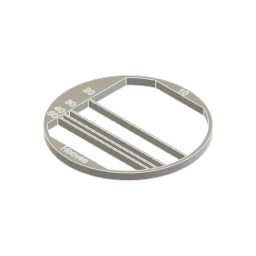
Range Finder-White Tail Deer v3 (Autodesk Fusion 360 design; units mm, degrees)
Autodesk Fusion 360 part; units mm, degrees
sketch "Sketch1" plane through (0, 0, 0) normal (0, 1, 0) x (1, 0, 0)
  circle A0 centre (0, 0) radius 57.15
  circle A1 centre (0, 0) radius 54.61
  dimension "d1" = 114.3
  dimension "d2" = 109.22
  constraint coincident A0.centre A1.centre
  constraint concentric A0 A1
  measures "d1" diameter of A0
  measures "d2" diameter of A1
extrude "Extrude1" add sketch "Sketch1" along normal blind 6.35
sketch "Sketch2" plane through (0, 6.35, 0) normal (0, 1, 0) x (-1, 0, 0)
  circle A0 centre (0, 0) radius 54.61
  circle A1 centre (0, 0) radius 57.15
  line L0 (0, 54.61) -> (0, 46.99)
  line L1 (0, 46.99) -> (27.8243, 46.99)
  line L2 (-27.8243, 46.99) -> (0, 46.99)
  dimension "d5" = 7.62
  constraint coincident A0 L0.start
  constraint vertical L0
  constraint coincident A0 L1.end
  constraint perpendicular L0 L1
  constraint coincident A0 L2.start
  constraint perpendicular L0 L2
  measures "d5" distance of L0.start L0.end
extrude "Extrude2" add sketch "Sketch2" against normal blind 6.35 contours A0 L0 L1 | A0 L0 L2
sketch "Sketch3" plane through (0, 6.35, 0) normal (0, 1, 0) x (-1, 0, 0)
  arc A0 (-27.8243, 46.99) -> (27.8243, 46.99) centre (0, 0) ccw
  line L0 (-27.8243, 46.99) -> (27.8243, 46.99)
  circle A1 centre (0, 0) radius 57.15
  line L1 (0, -49.53) -> (23.0007, -49.53)
  line L2 (0, -49.53) -> (-23.0007, -49.53)
  arc A2 (-23.0007, -49.53) -> (23.0007, -49.53) centre (0, 0) ccw
  line L3 (54.5858, -1.6242) -> (-54.5952, -1.27)
  line L4 (-52.0545, 16.51) -> (52.0545, 16.51)
  line L5 (0, 22.86) -> (49.5951, 22.86)
  line L6 (0, 22.86) -> (-49.5951, 22.86)
  line L7 (0, 27.686) -> (47.0716, 27.686)
  line L8 (0, 27.686) -> (-47.0716, 27.686)
  line L9 (0, 27.686) -> (0, 26.416)
  line L10 (0, 22.86) -> (0, 21.59)
  line L11 (0, 16.51) -> (0, 15.24)
  line L12 (-0.0047, -1.4471) -> (-0.0088, -2.7171)
  line L13 (-0.0088, -2.7171) -> (54.5333, -2.894)
  line L14 (-0.0088, -2.7171) -> (-54.5509, -2.5402)
  line L15 (0, 15.24) -> (52.4404, 15.24)
  line L16 (0, 15.24) -> (-52.4404, 15.24)
  line L17 (0, 21.59) -> (-50.161, 21.59)
  line L18 (0, 21.59) -> (50.161, 21.59)
  line L19 (0, 26.416) -> (47.7959, 26.416)
  line L20 (0, 26.416) -> (-47.7959, 26.416)
  dimension "d16" = 1.27
  dimension "d17" = 1.27
  dimension "d18" = 1.27
  dimension "d19" = 1.27
  constraint coincident A0 L1.end
  constraint coincident A0 L2.end
  constraint coincident A0 L3.end
  constraint coincident A0 L3.start
  constraint coincident A0 L4.end
  constraint coincident A0 L4.start
  constraint horizontal L4
  constraint coincident A0 L5.end
  constraint coincident A0 L6.end
  constraint coincident A0 L7.end
  constraint coincident A0 L8.end
  constraint perpendicular L7 L9
  constraint perpendicular L6 L10
  constraint midpoint L4 L11.start
  constraint perpendicular L4 L11
  constraint midpoint L3 L12.start
  constraint perpendicular L3 L12
  constraint coincident A0 L13.end
  constraint perpendicular L12 L13
  constraint coincident A0 L14.end
  constraint perpendicular L12 L14
  constraint coincident A0 L15.end
  constraint perpendicular L11 L15
  constraint coincident A0 L16.end
  constraint perpendicular L11 L16
  constraint coincident A0 L17.end
  constraint perpendicular L10 L17
  constraint coincident A0 L18.end
  constraint perpendicular L10 L18
  constraint coincident A0 L19.end
  constraint perpendicular L9 L19
  constraint perpendicular L9 L20
  constraint coincident A0 L20.end
  constraint horizontal L20
  measures "d16" distance of L7.start L9.end
  measures "d17" distance of L5.start L10.end
  measures "d18" distance of L11.start L11.end
  measures "d19" distance of L12.start L12.end
extrude "Extrude3" add sketch "Sketch3" against normal blind 6.35 contours A0 L8 L9 L20 | A0 L7 L9 L19 | A0 L6 L10 L17 | A0 L5 L10 L18 | A0 L4 L11 L16 | A0 L4 L11 L15 | A0 L3 L12 L14 | A0 L3 L12 L13 | A0 L1 L2 A2
sketch "Sketch4" plane through (0, 6.35, 0) normal (0, 1, 0) x (-1, 0, 0)
  arc A0 (-52.4404, 15.24) -> (-54.5952, -1.27) centre (0, 0) ccw
  line L0 (-52.4404, 15.24) -> (52.4404, 15.24)
  arc A1 (54.5858, -1.6242) -> (52.4404, 15.24) centre (0, 0) ccw
  line L1 (54.5858, -1.6242) -> (-54.5952, -1.27)
  arc A2 (-27.8243, 46.99) -> (-47.0716, 27.686) centre (0, 0) ccw
  line L2 (-27.8243, 46.99) -> (27.8243, 46.99)
  arc A3 (47.0716, 27.686) -> (27.8243, 46.99) centre (0, 0) ccw
  line L3 (47.0716, 27.686) -> (-47.0716, 27.686)
  arc A4 (-50.161, 21.59) -> (-52.0545, 16.51) centre (0, 0) ccw
  line L4 (-50.161, 21.59) -> (50.161, 21.59)
  arc A5 (52.0545, 16.51) -> (50.161, 21.59) centre (0, 0) ccw
  line L5 (52.0545, 16.51) -> (-52.0545, 16.51)
  line L6 (-47.7959, 26.416) -> (47.7959, 26.416)
  arc A6 (49.5951, 22.86) -> (47.7959, 26.416) centre (0, 0) ccw
  line L7 (49.5951, 22.86) -> (-49.5951, 22.86)
  arc A7 (-47.7959, 26.416) -> (-49.5951, 22.86) centre (0, 0) ccw
  line L8 (-54.5509, -2.5402) -> (54.5333, -2.894)
  arc A8 (23.0007, -49.53) -> (54.5333, -2.894) centre (0, 0) ccw
  line L9 (23.0007, -49.53) -> (-23.0007, -49.53)
  arc A9 (-54.5509, -2.5402) -> (-23.0007, -49.53) centre (0, 0) ccw
  circle A10 centre (0, 0) radius 57.15
  line L10 (20.3865, 53.4838) -> (-20.1396, 53.4838) construction
  line L11 (-20.1396, 53.4838) -> (-20.1396, 46.99) construction
  line L12 (-20.1396, 46.99) -> (20.3865, 46.99) construction
  line L13 (20.3865, 46.99) -> (20.3865, 53.4838) construction
  line L14 (6.9725, -49.53) -> (-6.8843, -49.53) construction
  line L15 (-6.8843, -49.53) -> (-6.8843, -56.7231) construction
  line L16 (-6.8843, -56.7231) -> (6.9725, -56.7231) construction
  line L17 (6.9725, -56.7231) -> (6.9725, -49.53) construction
  dimension "d22" = 5.08
  dimension "d24" = 5.08
  dimension "d25" = 0
  text T0 "Hooves" font "Arial" height 5.08 align centre middle in box 40.5261 x 6.4938 at (20.3865, 53.4838) x (-1, 0) y (0, -1) spacing 1
  text T1 "10" font "Arial" height 5.08 align centre middle in box 13.8568 x 7.1931 at (6.9725, -49.53) x (-1, 0) y (0, -1) spacing 1
  constraint coincident A10
  constraint coincident L2
  constraint coincident L9
extrude "Extrude4" cut sketch "Sketch4" against normal blind 1.27 text T1 T0
sketch "Sketch5" plane through (0, 6.35, 0) normal (0, 1, 0) x (-1, 0, 0)
  spline S0 degree 3 poles (5.2156, 52.8601) (5.458, 52.8423) (5.9273, 52.8079) (6.2896, 52.509) (6.4648, 52.3645) knots 0 0 0 0 0.070957 0.137381 0.137381 0.137381 0.137381
  spline S1 degree 3 poles (6.4648, 52.3645) (6.6035, 52.1699) (6.9064, 51.7448) (6.929, 51.2209) (6.9412, 50.9369) knots 0 0 0 0 0.070238 0.153394 0.153394 0.153394 0.153394
  spline S2 degree 3 poles (6.9412, 50.9369) (6.927, 50.6271) (6.9009, 50.0574) (6.5384, 49.6215) (6.3729, 49.4226) knots 0 0 0 0 0.090097 0.165714 0.165714 0.165714 0.165714
  spline S3 degree 3 poles (6.3729, 49.4226) (6.2035, 49.3033) (5.8563, 49.0591) (5.4325, 49.0291) (5.2156, 49.0137) knots 0 0 0 0 0.060949 0.124839 0.124839 0.124839 0.124839
  spline S4 degree 3 poles (5.2156, 49.0137) (4.9764, 49.0322) (4.51, 49.0682) (4.1502, 49.3659) (3.975, 49.5109) knots 0 0 0 0 0.070069 0.136601 0.136601 0.136601 0.136601
  spline S5 degree 3 poles (3.975, 49.5109) (3.8347, 49.701) (3.5343, 50.1079) (3.5076, 50.6148) (3.4934, 50.8849) knots 0 0 0 0 0.069362 0.148467 0.148467 0.148467 0.148467
  spline S6 degree 3 poles (3.4934, 50.8849) (3.4975, 51.0992) (3.505, 51.4847) (3.6445, 51.8432) (3.7065, 52.0024) knots 0 0 0 0 0.06368 0.114552 0.114552 0.114552 0.114552
  spline S7 degree 3 poles (3.7065, 52.0024) (3.7858, 52.1307) (3.945, 52.3881) (4.1992, 52.5524) (4.3267, 52.6348) knots 0 0 0 0 0.044639 0.089574 0.089574 0.089574 0.089574
  spline S8 degree 3 poles (4.3267, 52.6348) (4.4663, 52.7005) (4.7479, 52.8331) (5.0587, 52.851) (5.2156, 52.8601) knots 0 0 0 0 0.045807 0.092452 0.092452 0.092452 0.092452
  spline S9 degree 3 poles (-10.0036, 52.8601) (-9.7875, 52.854) (-9.3973, 52.843) (-9.0606, 52.6487) (-8.9104, 52.5621) knots 0 0 0 0 0.063634 0.114894 0.114894 0.114894 0.114894
  spline S10 degree 3 poles (-8.9104, 52.5621) (-8.7955, 52.4455) (-8.5515, 52.1979) (-8.4723, 51.8583) (-8.4304, 51.6784) knots 0 0 0 0 0.048133 0.102307 0.102307 0.102307 0.102307
  line L0 (-8.4304, 51.6784) -> (-9.0472, 51.5814)
  spline S11 degree 3 poles (-9.0472, 51.5814) (-9.07, 51.6958) (-9.1132, 51.913) (-9.2648, 52.0737) (-9.3366, 52.1497) knots 0 0 0 0 0.034191 0.06493 0.06493 0.06493 0.06493
  spline S12 degree 3 poles (-9.3366, 52.1497) (-9.4289, 52.2072) (-9.6312, 52.3332) (-9.8702, 52.3423) (-10.0002, 52.3472) knots 0 0 0 0 0.032083 0.070304 0.070304 0.070304 0.070304
  spline S13 degree 3 poles (-10.0002, 52.3472) (-10.1284, 52.3443) (-10.3567, 52.339) (-10.5521, 52.2231) (-10.6378, 52.1722) knots 0 0 0 0 0.037679 0.067104 0.067104 0.067104 0.067104
  spline S14 degree 3 poles (-10.6378, 52.1722) (-10.6984, 52.1131) (-10.8148, 51.9995) (-10.8357, 51.8387) (-10.8457, 51.7616) knots 0 0 0 0 0.024591 0.047243 0.047243 0.047243 0.047243
  spline S15 degree 3 poles (-10.8457, 51.7616) (-10.8377, 51.6947) (-10.8214, 51.5591) (-10.7156, 51.4727) (-10.662, 51.4289) knots 0 0 0 0 0.019436 0.039349 0.039349 0.039349 0.039349
  spline S16 degree 3 poles (-10.662, 51.4289) (-10.5881, 51.3958) (-10.3832, 51.3037) (-10.1644, 51.2512) (-10.0244, 51.2176) knots 0 0 0 0 0.024263 0.067292 0.067292 0.067292 0.067292
  spline S17 degree 3 poles (-10.0244, 51.2176) (-9.8292, 51.1687) (-9.506, 51.0877) (-9.196, 50.966) (-9.0732, 50.9178) knots 0 0 0 0 0.060291 0.099819 0.099819 0.099819 0.099819
  spline S18 degree 3 poles (-9.0732, 50.9178) (-8.991, 50.8728) (-8.8312, 50.7854) (-8.7235, 50.6389) (-8.6713, 50.5678) knots 0 0 0 0 0.027754 0.053876 0.053876 0.053876 0.053876
  spline S19 degree 3 poles (-8.6713, 50.5678) (-8.6314, 50.491) (-8.5509, 50.3361) (-8.5399, 50.1619) (-8.5344, 50.074) knots 0 0 0 0 0.025663 0.051747 0.051747 0.051747 0.051747
  spline S20 degree 3 poles (-8.5344, 50.074) (-8.5389, 49.9939) (-8.5479, 49.8349) (-8.6142, 49.6901) (-8.647, 49.6184) knots 0 0 0 0 0.02386 0.047308 0.047308 0.047308 0.047308
  spline S21 degree 3 poles (-8.647, 49.6184) (-8.688, 49.5514) (-8.7699, 49.4175) (-8.8924, 49.3193) (-8.9537, 49.2701) knots 0 0 0 0 0.023346 0.046717 0.046717 0.046717 0.046717
  spline S22 degree 3 poles (-8.9537, 49.2701) (-9.0099, 49.2347) (-9.134, 49.1567) (-9.2739, 49.1124) (-9.3505, 49.0882) knots 0 0 0 0 0.019852 0.043806 0.043806 0.043806 0.043806
  spline S23 degree 3 poles (-9.3505, 49.0882) (-9.4368, 49.0665) (-9.6137, 49.022) (-9.796, 49.0165) (-9.8893, 49.0137) knots 0 0 0 0 0.026625 0.054539 0.054539 0.054539 0.054539
  spline S24 degree 3 poles (-9.8893, 49.0137) (-10.026, 49.0177) (-10.2853, 49.0252) (-10.5328, 49.1021) (-10.6499, 49.1384) knots 0 0 0 0 0.040792 0.077397 0.077397 0.077397 0.077397
  spline S25 degree 3 poles (-10.6499, 49.1384) (-10.7496, 49.1807) (-10.9351, 49.2592) (-11.0706, 49.4076) (-11.1333, 49.4763) knots 0 0 0 0 0.032023 0.059594 0.059594 0.059594 0.059594
  spline S26 degree 3 poles (-11.1333, 49.4763) (-11.1819, 49.5575) (-11.2876, 49.7343) (-11.3269, 49.9368) (-11.3482, 50.0463) knots 0 0 0 0 0.028173 0.061329 0.061329 0.061329 0.061329
  line L1 (-11.3482, 50.0463) -> (-10.7383, 50.1295)
  spline S27 degree 3 poles (-10.7383, 50.1295) (-10.719, 50.0409) (-10.6817, 49.8694) (-10.5575, 49.7457) (-10.4974, 49.6859) knots 0 0 0 0 0.026561 0.051435 0.051435 0.051435 0.051435
  spline S28 degree 3 poles (-10.4974, 49.6859) (-10.4193, 49.6396) (-10.2464, 49.537) (-10.0448, 49.5302) (-9.9343, 49.5265) knots 0 0 0 0 0.026848 0.059363 0.059363 0.059363 0.059363
  spline S29 degree 3 poles (-9.9343, 49.5265) (-9.8088, 49.5276) (-9.5926, 49.5293) (-9.4013, 49.6274) (-9.321, 49.6686) knots 0 0 0 0 0.036989 0.063721 0.063721 0.063721 0.063721
  spline S30 degree 3 poles (-9.321, 49.6686) (-9.2675, 49.716) (-9.1663, 49.8055) (-9.1466, 49.9386) (-9.1373, 50.0013) knots 0 0 0 0 0.020676 0.039103 0.039103 0.039103 0.039103
  spline S31 degree 3 poles (-9.1373, 50.0013) (-9.1406, 50.0408) (-9.1471, 50.1201) (-9.1913, 50.1863) (-9.2136, 50.2196) knots 0 0 0 0 0.011678 0.023467 0.023467 0.023467 0.023467
  spline S32 degree 3 poles (-9.2136, 50.2196) (-9.2446, 50.2524) (-9.3126, 50.3243) (-9.4034, 50.3642) (-9.4527, 50.3859) knots 0 0 0 0 0.013422 0.029388 0.029388 0.029388 0.029388
  spline S33 degree 3 poles (-9.4527, 50.3859) (-9.5141, 50.4053) (-9.6965, 50.4627) (-9.8812, 50.5124) (-10.0036, 50.5453) knots 0 0 0 0 0.019318 0.057361 0.057361 0.057361 0.057361
  spline S34 degree 3 poles (-10.0036, 50.5453) (-10.192, 50.5953) (-10.5042, 50.6782) (-10.8071, 50.7903) (-10.9271, 50.8347) knots 0 0 0 0 0.058433 0.096821 0.096821 0.096821 0.096821
  spline S35 degree 3 poles (-10.9271, 50.8347) (-11.009, 50.8756) (-11.1693, 50.9557) (-11.2824, 51.0944) (-11.3378, 51.1621) knots 0 0 0 0 0.027129 0.053055 0.053055 0.053055 0.053055
  spline S36 degree 3 poles (-11.3378, 51.1621) (-11.3812, 51.2406) (-11.4729, 51.4064) (-11.482, 51.596) (-11.4868, 51.6958) knots 0 0 0 0 0.02655 0.056067 0.056067 0.056067 0.056067
  spline S37 degree 3 poles (-11.4868, 51.6958) (-11.4787, 51.7989) (-11.4624, 52.0083) (-11.3579, 52.1906) (-11.3048, 52.2831) knots 0 0 0 0 0.030617 0.062177 0.062177 0.062177 0.062177
  spline S38 degree 3 poles (-11.3048, 52.2831) (-11.2357, 52.3705) (-11.0925, 52.5514) (-10.8864, 52.6555) (-10.7799, 52.7093) knots 0 0 0 0 0.033024 0.068346 0.068346 0.068346 0.068346
  spline S39 degree 3 poles (-10.7799, 52.7093) (-10.6592, 52.7533) (-10.4086, 52.8446) (-10.142, 52.8548) (-10.0036, 52.8601) knots 0 0 0 0 0.038266 0.079502 0.079502 0.079502 0.079502
  spline S40 degree 3 poles (-6.282, 52.3472) (-6.3907, 52.3408) (-6.6008, 52.3284) (-6.7808, 52.2196) (-6.8676, 52.167) knots 0 0 0 0 0.032111 0.062098 0.062098 0.062098 0.062098
  spline S41 degree 3 poles (-6.8676, 52.167) (-6.946, 52.0931) (-7.1175, 51.9311) (-7.2048, 51.7113) (-7.2523, 51.5918) knots 0 0 0 0 0.031936 0.069943 0.069943 0.069943 0.069943
  line L2 (-7.2523, 51.5918) -> (-7.8968, 51.6715)
  spline S42 degree 3 poles (-7.8968, 51.6715) (-7.8376, 51.8474) (-7.723, 52.1877) (-7.4594, 52.4307) (-7.332, 52.5482) knots 0 0 0 0 0.054669 0.105795 0.105795 0.105795 0.105795
  spline S43 degree 3 poles (-7.332, 52.5482) (-7.1794, 52.6391) (-6.8555, 52.832) (-6.4782, 52.8504) (-6.2785, 52.8601) knots 0 0 0 0 0.052457 0.111364 0.111364 0.111364 0.111364
  spline S44 degree 3 poles (-6.2785, 52.8601) (-6.0274, 52.8434) (-5.547, 52.8116) (-5.1754, 52.5078) (-4.9982, 52.3628) knots 0 0 0 0 0.073439 0.140438 0.140438 0.140438 0.140438
  spline S45 degree 3 poles (-4.9982, 52.3628) (-4.8604, 52.1706) (-4.5628, 51.7555) (-4.5383, 51.2432) (-4.5251, 50.9681) knots 0 0 0 0 0.069472 0.150087 0.150087 0.150087 0.150087
  spline S46 degree 3 poles (-4.5251, 50.9681) (-4.5381, 50.6838) (-4.5622, 50.1561) (-4.8641, 49.7253) (-5.0033, 49.5265) knots 0 0 0 0 0.083334 0.154684 0.154684 0.154684 0.154684
  spline S47 degree 3 poles (-5.0033, 49.5265) (-5.1775, 49.377) (-5.5342, 49.0706) (-6.0036, 49.033) (-6.2439, 49.0137) knots 0 0 0 0 0.067053 0.137362 0.137362 0.137362 0.137362
  spline S48 degree 3 poles (-6.2439, 49.0137) (-6.477, 49.0328) (-6.9338, 49.0704) (-7.2802, 49.3696) (-7.4498, 49.5161) knots 0 0 0 0 0.068218 0.133689 0.133689 0.133689 0.133689
  spline S49 degree 3 poles (-7.4498, 49.5161) (-7.586, 49.711) (-7.8815, 50.1337) (-7.905, 50.6511) (-7.9176, 50.9299) knots 0 0 0 0 0.06991 0.151663 0.151663 0.151663 0.151663
  spline S50 degree 3 poles (-7.9176, 50.9299) (-7.9174, 50.9531) (-7.9168, 51.0085) (-7.9151, 51.0639) (-7.9141, 51.0963) knots 0 0 0 0 0.006931 0.016637 0.016637 0.016637 0.016637
  line L3 (-7.9141, 51.0963) -> (-5.1697, 51.0963)
  spline S51 degree 3 poles (-5.1697, 51.0963) (-5.1877, 51.2811) (-5.221, 51.622) (-5.4211, 51.8984) (-5.5127, 52.025) knots 0 0 0 0 0.054521 0.100594 0.100594 0.100594 0.100594
  spline S52 degree 3 poles (-5.5127, 52.025) (-5.6226, 52.1189) (-5.8443, 52.3087) (-6.1352, 52.3343) (-6.282, 52.3472) knots 0 0 0 0 0.042249 0.085285 0.085285 0.085285 0.085285
  spline S53 degree 3 poles (-1.6902, -50.4999) (-1.4604, -50.5195) (-1.012, -50.5578) (-0.6922, -50.873) (-0.5363, -51.0266) knots 0 0 0 0 0.066888 0.130463 0.130463 0.130463 0.130463
  spline S54 degree 3 poles (-0.5363, -51.0266) (-0.3906, -51.299) (-0.0475, -51.9401) (-0.0388, -52.6713) (-0.0338, -53.0919) knots 0 0 0 0 0.091462 0.215289 0.215289 0.215289 0.215289
  spline S55 degree 3 poles (-0.0338, -53.0919) (-0.0375, -53.3645) (-0.0441, -53.8554) (-0.1653, -54.3307) (-0.2192, -54.5421) knots 0 0 0 0 0.081435 0.146651 0.146651 0.146651 0.146651
  spline S56 degree 3 poles (-0.2192, -54.5421) (-0.2849, -54.7116) (-0.4094, -55.0331) (-0.6544, -55.275) (-0.7702, -55.3893) knots 0 0 0 0 0.053825 0.102088 0.102088 0.102088 0.102088
  spline S57 degree 3 poles (-0.7702, -55.3893) (-0.9037, -55.4762) (-1.1829, -55.6579) (-1.5162, -55.6772) (-1.6902, -55.6873) knots 0 0 0 0 0.046942 0.098208 0.098208 0.098208 0.098208
  spline S58 degree 3 poles (-1.6902, -55.6873) (-1.82, -55.6817) (-2.0694, -55.6708) (-2.2979, -55.5707) (-2.4075, -55.5227) knots 0 0 0 0 0.038597 0.074161 0.074161 0.074161 0.074161
  spline S59 degree 3 poles (-2.4075, -55.5227) (-2.5063, -55.4611) (-2.7068, -55.3359) (-2.8462, -55.1449) (-2.9169, -55.048) knots 0 0 0 0 0.034592 0.070208 0.070208 0.070208 0.070208
  spline S60 degree 3 poles (-2.9169, -55.048) (-2.9812, -54.9353) (-3.1174, -54.6966) (-3.1925, -54.4321) (-3.2322, -54.2926) knots 0 0 0 0 0.038787 0.082125 0.082125 0.082125 0.082125
  spline S61 degree 3 poles (-3.2322, -54.2926) (-3.2654, -54.1188) (-3.3412, -53.7224) (-3.3446, -53.3186) (-3.3466, -53.0919) knots 0 0 0 0 0.05298 0.120829 0.120829 0.120829 0.120829
  spline S62 degree 3 poles (-3.3466, -53.0919) (-3.3429, -52.821) (-3.3362, -52.3325) (-3.2163, -51.8594) (-3.1629, -51.6486) knots 0 0 0 0 0.080913 0.145932 0.145932 0.145932 0.145932
  spline S63 degree 3 poles (-3.1629, -51.6486) (-3.0977, -51.479) (-2.9739, -51.157) (-2.7294, -50.9144) (-2.6137, -50.7996) knots 0 0 0 0 0.053809 0.10214 0.10214 0.10214 0.10214
  spline S64 degree 3 poles (-2.6137, -50.7996) (-2.4799, -50.7123) (-2.1998, -50.5293) (-1.8651, -50.51) (-1.6902, -50.4999) knots 0 0 0 0 0.04708 0.09861 0.09861 0.09861 0.09861
  line L4 (1.9656, -55.6873) -> (1.5636, -55.6873)
  line L5 (1.5636, -55.6873) -> (1.5636, -50.5865)
  line L6 (1.5636, -50.5865) -> (2.1874, -50.5865)
  line L7 (2.1874, -50.5865) -> (2.1874, -54.5611)
  spline S65 degree 3 poles (2.1874, -54.5611) (2.2724, -54.4871) (2.4567, -54.3267) (2.6656, -54.1998) (2.7782, -54.1314) knots 0 0 0 0 0.033753 0.073172 0.073172 0.073172 0.073172
  spline S66 degree 3 poles (2.7782, -54.1314) (2.8925, -54.066) (3.1046, -53.9446) (3.3306, -53.8519) (3.4348, -53.8092) knots 0 0 0 0 0.039461 0.073217 0.073217 0.073217 0.073217
  line L8 (3.4348, -53.8092) -> (3.4348, -54.4121)
  spline S67 degree 3 poles (3.4348, -54.4121) (3.2676, -54.497) (2.9411, -54.6626) (2.6581, -54.8949) (2.52, -55.0081) knots 0 0 0 0 0.056073 0.109474 0.109474 0.109474 0.109474
  spline S68 degree 3 poles (2.52, -55.0081) (2.4022, -55.1179) (2.1861, -55.3192) (2.0345, -55.5723) (1.9656, -55.6873) knots 0 0 0 0 0.048031 0.088061 0.088061 0.088061 0.088061
  line L9 (-4.1821, 49.0969) -> (-2.7891, 52.7769)
  line L10 (-2.7891, 52.7769) -> (-2.2069, 52.7769)
  line L11 (-2.2069, 52.7769) -> (-0.807, 49.0969)
  line L12 (-0.807, 49.0969) -> (-1.4654, 49.0969)
  line L13 (-1.4654, 49.0969) -> (-2.2554, 51.3007)
  spline S69 degree 3 poles (-2.2554, 51.3007) (-2.2975, 51.4217) (-2.3828, 51.6667) (-2.4547, 51.916) (-2.4911, 52.0423) knots 0 0 0 0 0.038408 0.077822 0.077822 0.077822 0.077822
  spline S70 degree 3 poles (-2.4911, 52.0423) (-2.5234, 51.9352) (-2.5946, 51.6998) (-2.6779, 51.4684) (-2.7232, 51.3423) knots 0 0 0 0 0.033566 0.073758 0.073758 0.073758 0.073758
  line L14 (-2.7232, 51.3423) -> (-3.541, 49.0969)
  line L15 (-3.541, 49.0969) -> (-4.1821, 49.0969)
  spline S71 degree 3 poles (1.2687, 52.8601) (1.5111, 52.8423) (1.9804, 52.8079) (2.3427, 52.509) (2.5179, 52.3645) knots 0 0 0 0 0.070957 0.137381 0.137381 0.137381 0.137381
  spline S72 degree 3 poles (2.5179, 52.3645) (2.6566, 52.1699) (2.9595, 51.7448) (2.9821, 51.2209) (2.9944, 50.9369) knots 0 0 0 0 0.070238 0.153394 0.153394 0.153394 0.153394
  spline S73 degree 3 poles (2.9944, 50.9369) (2.9801, 50.6271) (2.954, 50.0574) (2.5915, 49.6215) (2.4261, 49.4226) knots 0 0 0 0 0.090097 0.165714 0.165714 0.165714 0.165714
  spline S74 degree 3 poles (2.4261, 49.4226) (2.2566, 49.3033) (1.9095, 49.0591) (1.4856, 49.0291) (1.2687, 49.0137) knots 0 0 0 0 0.060949 0.124838 0.124838 0.124838 0.124838
  spline S75 degree 3 poles (1.2687, 49.0137) (1.0295, 49.0322) (0.5631, 49.0682) (0.2034, 49.3659) (0.0281, 49.5109) knots 0 0 0 0 0.070069 0.136601 0.136601 0.136601 0.136601
  spline S76 degree 3 poles (0.0281, 49.5109) (-0.1122, 49.701) (-0.4125, 50.1079) (-0.4393, 50.6148) (-0.4535, 50.8849) knots 0 0 0 0 0.069362 0.148467 0.148467 0.148467 0.148467
  spline S77 degree 3 poles (-0.4535, 50.8849) (-0.4494, 51.0992) (-0.4419, 51.4847) (-0.3024, 51.8432) (-0.2404, 52.0024) knots 0 0 0 0 0.06368 0.114552 0.114552 0.114552 0.114552
  spline S78 degree 3 poles (-0.2404, 52.0024) (-0.1611, 52.1307) (-0.0019, 52.3881) (0.2523, 52.5524) (0.3799, 52.6348) knots 0 0 0 0 0.044639 0.089574 0.089574 0.089574 0.089574
  spline S79 degree 3 poles (0.3799, 52.6348) (0.5194, 52.7005) (0.801, 52.8331) (1.1119, 52.851) (1.2687, 52.8601) knots 0 0 0 0 0.045808 0.092453 0.092453 0.092453 0.092453
  line L16 (11.0614, 50.3824) -> (11.0614, 52.7769)
  line L17 (11.0614, 52.7769) -> (11.7336, 52.7769)
  line L18 (11.7336, 52.7769) -> (11.7336, 47.6969)
  line L19 (11.7336, 47.6969) -> (11.0614, 47.6969)
  line L20 (11.0614, 47.6969) -> (11.0614, 49.783)
  line L21 (11.0614, 49.783) -> (8.4209, 49.783)
  line L22 (8.4209, 49.783) -> (8.4209, 47.6969)
  line L23 (8.4209, 47.6969) -> (7.7486, 47.6969)
  line L24 (7.7486, 47.6969) -> (7.7486, 52.7769)
  line L25 (7.7486, 52.7769) -> (8.4209, 52.7769)
  line L26 (8.4209, 52.7769) -> (8.4209, 50.3824)
  line L27 (8.4209, 50.3824) -> (11.0614, 50.3824)
  arc A0 (-52.4404, 15.24) -> (-54.5952, -1.27) centre (0, 0) ccw
  line L28 (-52.4404, 15.24) -> (52.4404, 15.24)
  arc A1 (54.5858, -1.6242) -> (52.4404, 15.24) centre (0, 0) ccw
  line L29 (54.5858, -1.6242) -> (-54.5952, -1.27)
  arc A2 (-27.8243, 46.99) -> (-47.0716, 27.686) centre (0, 0) ccw
  line L30 (-27.8243, 46.99) -> (27.8243, 46.99)
  arc A3 (47.0716, 27.686) -> (27.8243, 46.99) centre (0, 0) ccw
  line L31 (47.0716, 27.686) -> (-47.0716, 27.686)
  arc A4 (-50.161, 21.59) -> (-52.0545, 16.51) centre (0, 0) ccw
  line L32 (-50.161, 21.59) -> (50.161, 21.59)
  arc A5 (52.0545, 16.51) -> (50.161, 21.59) centre (0, 0) ccw
  line L33 (52.0545, 16.51) -> (-52.0545, 16.51)
  line L34 (-47.7959, 26.416) -> (47.7959, 26.416)
  arc A6 (49.5951, 22.86) -> (47.7959, 26.416) centre (0, 0) ccw
  line L35 (49.5951, 22.86) -> (-49.5951, 22.86)
  arc A7 (-47.7959, 26.416) -> (-49.5951, 22.86) centre (0, 0) ccw
  line L36 (-54.5509, -2.5402) -> (54.5333, -2.894)
  arc A8 (23.0007, -49.53) -> (54.5333, -2.894) centre (0, 0) ccw
  line L37 (23.0007, -49.53) -> (-23.0007, -49.53)
  arc A9 (-54.5509, -2.5402) -> (-23.0007, -49.53) centre (0, 0) ccw
  circle A10 centre (0, 0) radius 57.15
  line L38 (47.0716, 27.686) -> (39.4516, 27.686)
  line L39 (39.4516, 37.7601) -> (39.4516, -37.7601)
  dimension "d28" = 7.62
  constraint coincident A3.start L31.start
  constraint parallel L31 L38
  constraint coincident A3 L39.start
  constraint coincident A8 L39.end
  constraint vertical L39
  measures "d28" distance of A3.start L38.end
extrude "Extrude5" add sketch "Sketch5" against normal blind 6.35 contours L28 A1 L29 L39 | A3 L31 L38 L39 | L32 A5 L33 L39 | L34 A6 L35 L39 | L36 A8 L39
sketch "Sketch6" plane through (0, 6.35, 0) normal (0, 1, 0) x (-1, 0, 0)
  spline S0 degree 3 poles (5.2156, 52.8601) (5.458, 52.8423) (5.9273, 52.8079) (6.2896, 52.509) (6.4648, 52.3645) knots 0 0 0 0 0.070957 0.137381 0.137381 0.137381 0.137381
  spline S1 degree 3 poles (6.4648, 52.3645) (6.6035, 52.1699) (6.9064, 51.7448) (6.929, 51.2209) (6.9412, 50.9369) knots 0 0 0 0 0.070238 0.153394 0.153394 0.153394 0.153394
  spline S2 degree 3 poles (6.9412, 50.9369) (6.927, 50.6271) (6.9009, 50.0574) (6.5384, 49.6215) (6.3729, 49.4226) knots 0 0 0 0 0.090097 0.165714 0.165714 0.165714 0.165714
  spline S3 degree 3 poles (6.3729, 49.4226) (6.2035, 49.3033) (5.8563, 49.0591) (5.4325, 49.0291) (5.2156, 49.0137) knots 0 0 0 0 0.060949 0.124839 0.124839 0.124839 0.124839
  spline S4 degree 3 poles (5.2156, 49.0137) (4.9764, 49.0322) (4.51, 49.0682) (4.1502, 49.3659) (3.975, 49.5109) knots 0 0 0 0 0.070069 0.136601 0.136601 0.136601 0.136601
  spline S5 degree 3 poles (3.975, 49.5109) (3.8347, 49.701) (3.5343, 50.1079) (3.5076, 50.6148) (3.4934, 50.8849) knots 0 0 0 0 0.069362 0.148467 0.148467 0.148467 0.148467
  spline S6 degree 3 poles (3.4934, 50.8849) (3.4975, 51.0992) (3.505, 51.4847) (3.6445, 51.8432) (3.7065, 52.0024) knots 0 0 0 0 0.06368 0.114552 0.114552 0.114552 0.114552
  spline S7 degree 3 poles (3.7065, 52.0024) (3.7858, 52.1307) (3.945, 52.3881) (4.1992, 52.5524) (4.3267, 52.6348) knots 0 0 0 0 0.044639 0.089574 0.089574 0.089574 0.089574
  spline S8 degree 3 poles (4.3267, 52.6348) (4.4663, 52.7005) (4.7479, 52.8331) (5.0587, 52.851) (5.2156, 52.8601) knots 0 0 0 0 0.045807 0.092452 0.092452 0.092452 0.092452
  spline S9 degree 3 poles (-10.0036, 52.8601) (-9.7875, 52.854) (-9.3973, 52.843) (-9.0606, 52.6487) (-8.9104, 52.5621) knots 0 0 0 0 0.063634 0.114894 0.114894 0.114894 0.114894
  spline S10 degree 3 poles (-8.9104, 52.5621) (-8.7955, 52.4455) (-8.5515, 52.1979) (-8.4723, 51.8583) (-8.4304, 51.6784) knots 0 0 0 0 0.048133 0.102307 0.102307 0.102307 0.102307
  line L0 (-8.4304, 51.6784) -> (-9.0472, 51.5814)
  spline S11 degree 3 poles (-9.0472, 51.5814) (-9.07, 51.6958) (-9.1132, 51.913) (-9.2648, 52.0737) (-9.3366, 52.1497) knots 0 0 0 0 0.034191 0.06493 0.06493 0.06493 0.06493
  spline S12 degree 3 poles (-9.3366, 52.1497) (-9.4289, 52.2072) (-9.6312, 52.3332) (-9.8702, 52.3423) (-10.0002, 52.3472) knots 0 0 0 0 0.032083 0.070304 0.070304 0.070304 0.070304
  spline S13 degree 3 poles (-10.0002, 52.3472) (-10.1284, 52.3443) (-10.3567, 52.339) (-10.5521, 52.2231) (-10.6378, 52.1722) knots 0 0 0 0 0.037679 0.067104 0.067104 0.067104 0.067104
  spline S14 degree 3 poles (-10.6378, 52.1722) (-10.6984, 52.1131) (-10.8148, 51.9995) (-10.8357, 51.8387) (-10.8457, 51.7616) knots 0 0 0 0 0.024591 0.047243 0.047243 0.047243 0.047243
  spline S15 degree 3 poles (-10.8457, 51.7616) (-10.8377, 51.6947) (-10.8214, 51.5591) (-10.7156, 51.4727) (-10.662, 51.4289) knots 0 0 0 0 0.019436 0.039349 0.039349 0.039349 0.039349
  spline S16 degree 3 poles (-10.662, 51.4289) (-10.5881, 51.3958) (-10.3832, 51.3037) (-10.1644, 51.2512) (-10.0244, 51.2176) knots 0 0 0 0 0.024263 0.067292 0.067292 0.067292 0.067292
  spline S17 degree 3 poles (-10.0244, 51.2176) (-9.8292, 51.1687) (-9.506, 51.0877) (-9.196, 50.966) (-9.0732, 50.9178) knots 0 0 0 0 0.060291 0.099819 0.099819 0.099819 0.099819
  spline S18 degree 3 poles (-9.0732, 50.9178) (-8.991, 50.8728) (-8.8312, 50.7854) (-8.7235, 50.6389) (-8.6713, 50.5678) knots 0 0 0 0 0.027754 0.053876 0.053876 0.053876 0.053876
  spline S19 degree 3 poles (-8.6713, 50.5678) (-8.6314, 50.491) (-8.5509, 50.3361) (-8.5399, 50.1619) (-8.5344, 50.074) knots 0 0 0 0 0.025663 0.051747 0.051747 0.051747 0.051747
  spline S20 degree 3 poles (-8.5344, 50.074) (-8.5389, 49.9939) (-8.5479, 49.8349) (-8.6142, 49.6901) (-8.647, 49.6184) knots 0 0 0 0 0.02386 0.047308 0.047308 0.047308 0.047308
  spline S21 degree 3 poles (-8.647, 49.6184) (-8.688, 49.5514) (-8.7699, 49.4175) (-8.8924, 49.3193) (-8.9537, 49.2701) knots 0 0 0 0 0.023346 0.046717 0.046717 0.046717 0.046717
  spline S22 degree 3 poles (-8.9537, 49.2701) (-9.0099, 49.2347) (-9.134, 49.1567) (-9.2739, 49.1124) (-9.3505, 49.0882) knots 0 0 0 0 0.019852 0.043806 0.043806 0.043806 0.043806
  spline S23 degree 3 poles (-9.3505, 49.0882) (-9.4368, 49.0665) (-9.6137, 49.022) (-9.796, 49.0165) (-9.8893, 49.0137) knots 0 0 0 0 0.026625 0.054539 0.054539 0.054539 0.054539
  spline S24 degree 3 poles (-9.8893, 49.0137) (-10.026, 49.0177) (-10.2853, 49.0252) (-10.5328, 49.1021) (-10.6499, 49.1384) knots 0 0 0 0 0.040792 0.077397 0.077397 0.077397 0.077397
  spline S25 degree 3 poles (-10.6499, 49.1384) (-10.7496, 49.1807) (-10.9351, 49.2592) (-11.0706, 49.4076) (-11.1333, 49.4763) knots 0 0 0 0 0.032023 0.059594 0.059594 0.059594 0.059594
  spline S26 degree 3 poles (-11.1333, 49.4763) (-11.1819, 49.5575) (-11.2876, 49.7343) (-11.3269, 49.9368) (-11.3482, 50.0463) knots 0 0 0 0 0.028173 0.061329 0.061329 0.061329 0.061329
  line L1 (-11.3482, 50.0463) -> (-10.7383, 50.1295)
  spline S27 degree 3 poles (-10.7383, 50.1295) (-10.719, 50.0409) (-10.6817, 49.8694) (-10.5575, 49.7457) (-10.4974, 49.6859) knots 0 0 0 0 0.026561 0.051435 0.051435 0.051435 0.051435
  spline S28 degree 3 poles (-10.4974, 49.6859) (-10.4193, 49.6396) (-10.2464, 49.537) (-10.0448, 49.5302) (-9.9343, 49.5265) knots 0 0 0 0 0.026848 0.059363 0.059363 0.059363 0.059363
  spline S29 degree 3 poles (-9.9343, 49.5265) (-9.8088, 49.5276) (-9.5926, 49.5293) (-9.4013, 49.6274) (-9.321, 49.6686) knots 0 0 0 0 0.036989 0.063721 0.063721 0.063721 0.063721
  spline S30 degree 3 poles (-9.321, 49.6686) (-9.2675, 49.716) (-9.1663, 49.8055) (-9.1466, 49.9386) (-9.1373, 50.0013) knots 0 0 0 0 0.020676 0.039103 0.039103 0.039103 0.039103
  spline S31 degree 3 poles (-9.1373, 50.0013) (-9.1406, 50.0408) (-9.1471, 50.1201) (-9.1913, 50.1863) (-9.2136, 50.2196) knots 0 0 0 0 0.011678 0.023467 0.023467 0.023467 0.023467
  spline S32 degree 3 poles (-9.2136, 50.2196) (-9.2446, 50.2524) (-9.3126, 50.3243) (-9.4034, 50.3642) (-9.4527, 50.3859) knots 0 0 0 0 0.013422 0.029388 0.029388 0.029388 0.029388
  spline S33 degree 3 poles (-9.4527, 50.3859) (-9.5141, 50.4053) (-9.6965, 50.4627) (-9.8812, 50.5124) (-10.0036, 50.5453) knots 0 0 0 0 0.019318 0.057361 0.057361 0.057361 0.057361
  spline S34 degree 3 poles (-10.0036, 50.5453) (-10.192, 50.5953) (-10.5042, 50.6782) (-10.8071, 50.7903) (-10.9271, 50.8347) knots 0 0 0 0 0.058433 0.096821 0.096821 0.096821 0.096821
  spline S35 degree 3 poles (-10.9271, 50.8347) (-11.009, 50.8756) (-11.1693, 50.9557) (-11.2824, 51.0944) (-11.3378, 51.1621) knots 0 0 0 0 0.027129 0.053055 0.053055 0.053055 0.053055
  spline S36 degree 3 poles (-11.3378, 51.1621) (-11.3812, 51.2406) (-11.4729, 51.4064) (-11.482, 51.596) (-11.4868, 51.6958) knots 0 0 0 0 0.02655 0.056067 0.056067 0.056067 0.056067
  spline S37 degree 3 poles (-11.4868, 51.6958) (-11.4787, 51.7989) (-11.4624, 52.0083) (-11.3579, 52.1906) (-11.3048, 52.2831) knots 0 0 0 0 0.030617 0.062177 0.062177 0.062177 0.062177
  spline S38 degree 3 poles (-11.3048, 52.2831) (-11.2357, 52.3705) (-11.0925, 52.5514) (-10.8864, 52.6555) (-10.7799, 52.7093) knots 0 0 0 0 0.033024 0.068346 0.068346 0.068346 0.068346
  spline S39 degree 3 poles (-10.7799, 52.7093) (-10.6592, 52.7533) (-10.4086, 52.8446) (-10.142, 52.8548) (-10.0036, 52.8601) knots 0 0 0 0 0.038266 0.079502 0.079502 0.079502 0.079502
  spline S40 degree 3 poles (-6.282, 52.3472) (-6.3907, 52.3408) (-6.6008, 52.3284) (-6.7808, 52.2196) (-6.8676, 52.167) knots 0 0 0 0 0.032111 0.062098 0.062098 0.062098 0.062098
  spline S41 degree 3 poles (-6.8676, 52.167) (-6.946, 52.0931) (-7.1175, 51.9311) (-7.2048, 51.7113) (-7.2523, 51.5918) knots 0 0 0 0 0.031936 0.069943 0.069943 0.069943 0.069943
  line L2 (-7.2523, 51.5918) -> (-7.8968, 51.6715)
  spline S42 degree 3 poles (-7.8968, 51.6715) (-7.8376, 51.8474) (-7.723, 52.1877) (-7.4594, 52.4307) (-7.332, 52.5482) knots 0 0 0 0 0.054669 0.105795 0.105795 0.105795 0.105795
  spline S43 degree 3 poles (-7.332, 52.5482) (-7.1794, 52.6391) (-6.8555, 52.832) (-6.4782, 52.8504) (-6.2785, 52.8601) knots 0 0 0 0 0.052457 0.111364 0.111364 0.111364 0.111364
  spline S44 degree 3 poles (-6.2785, 52.8601) (-6.0274, 52.8434) (-5.547, 52.8116) (-5.1754, 52.5078) (-4.9982, 52.3628) knots 0 0 0 0 0.073439 0.140438 0.140438 0.140438 0.140438
  spline S45 degree 3 poles (-4.9982, 52.3628) (-4.8604, 52.1706) (-4.5628, 51.7555) (-4.5383, 51.2432) (-4.5251, 50.9681) knots 0 0 0 0 0.069472 0.150087 0.150087 0.150087 0.150087
  spline S46 degree 3 poles (-4.5251, 50.9681) (-4.5381, 50.6838) (-4.5622, 50.1561) (-4.8641, 49.7253) (-5.0033, 49.5265) knots 0 0 0 0 0.083334 0.154684 0.154684 0.154684 0.154684
  spline S47 degree 3 poles (-5.0033, 49.5265) (-5.1775, 49.377) (-5.5342, 49.0706) (-6.0036, 49.033) (-6.2439, 49.0137) knots 0 0 0 0 0.067053 0.137362 0.137362 0.137362 0.137362
  spline S48 degree 3 poles (-6.2439, 49.0137) (-6.477, 49.0328) (-6.9338, 49.0704) (-7.2802, 49.3696) (-7.4498, 49.5161) knots 0 0 0 0 0.068218 0.133689 0.133689 0.133689 0.133689
  spline S49 degree 3 poles (-7.4498, 49.5161) (-7.586, 49.711) (-7.8815, 50.1337) (-7.905, 50.6511) (-7.9176, 50.9299) knots 0 0 0 0 0.06991 0.151663 0.151663 0.151663 0.151663
  spline S50 degree 3 poles (-7.9176, 50.9299) (-7.9174, 50.9531) (-7.9168, 51.0085) (-7.9151, 51.0639) (-7.9141, 51.0963) knots 0 0 0 0 0.006931 0.016637 0.016637 0.016637 0.016637
  line L3 (-7.9141, 51.0963) -> (-5.1697, 51.0963)
  spline S51 degree 3 poles (-5.1697, 51.0963) (-5.1877, 51.2811) (-5.221, 51.622) (-5.4211, 51.8984) (-5.5127, 52.025) knots 0 0 0 0 0.054521 0.100594 0.100594 0.100594 0.100594
  spline S52 degree 3 poles (-5.5127, 52.025) (-5.6226, 52.1189) (-5.8443, 52.3087) (-6.1352, 52.3343) (-6.282, 52.3472) knots 0 0 0 0 0.042249 0.085285 0.085285 0.085285 0.085285
  spline S53 degree 3 poles (-1.6902, -50.4999) (-1.4604, -50.5195) (-1.012, -50.5578) (-0.6922, -50.873) (-0.5363, -51.0266) knots 0 0 0 0 0.066888 0.130463 0.130463 0.130463 0.130463
  spline S54 degree 3 poles (-0.5363, -51.0266) (-0.3906, -51.299) (-0.0475, -51.9401) (-0.0388, -52.6713) (-0.0338, -53.0919) knots 0 0 0 0 0.091462 0.215289 0.215289 0.215289 0.215289
  spline S55 degree 3 poles (-0.0338, -53.0919) (-0.0375, -53.3645) (-0.0441, -53.8554) (-0.1653, -54.3307) (-0.2192, -54.5421) knots 0 0 0 0 0.081435 0.146651 0.146651 0.146651 0.146651
  spline S56 degree 3 poles (-0.2192, -54.5421) (-0.2849, -54.7116) (-0.4094, -55.0331) (-0.6544, -55.275) (-0.7702, -55.3893) knots 0 0 0 0 0.053825 0.102088 0.102088 0.102088 0.102088
  spline S57 degree 3 poles (-0.7702, -55.3893) (-0.9037, -55.4762) (-1.1829, -55.6579) (-1.5162, -55.6772) (-1.6902, -55.6873) knots 0 0 0 0 0.046942 0.098208 0.098208 0.098208 0.098208
  spline S58 degree 3 poles (-1.6902, -55.6873) (-1.82, -55.6817) (-2.0694, -55.6708) (-2.2979, -55.5707) (-2.4075, -55.5227) knots 0 0 0 0 0.038597 0.074161 0.074161 0.074161 0.074161
  spline S59 degree 3 poles (-2.4075, -55.5227) (-2.5063, -55.4611) (-2.7068, -55.3359) (-2.8462, -55.1449) (-2.9169, -55.048) knots 0 0 0 0 0.034592 0.070208 0.070208 0.070208 0.070208
  spline S60 degree 3 poles (-2.9169, -55.048) (-2.9812, -54.9353) (-3.1174, -54.6966) (-3.1925, -54.4321) (-3.2322, -54.2926) knots 0 0 0 0 0.038787 0.082125 0.082125 0.082125 0.082125
  spline S61 degree 3 poles (-3.2322, -54.2926) (-3.2654, -54.1188) (-3.3412, -53.7224) (-3.3446, -53.3186) (-3.3466, -53.0919) knots 0 0 0 0 0.05298 0.120829 0.120829 0.120829 0.120829
  spline S62 degree 3 poles (-3.3466, -53.0919) (-3.3429, -52.821) (-3.3362, -52.3325) (-3.2163, -51.8594) (-3.1629, -51.6486) knots 0 0 0 0 0.080913 0.145932 0.145932 0.145932 0.145932
  spline S63 degree 3 poles (-3.1629, -51.6486) (-3.0977, -51.479) (-2.9739, -51.157) (-2.7294, -50.9144) (-2.6137, -50.7996) knots 0 0 0 0 0.053809 0.10214 0.10214 0.10214 0.10214
  spline S64 degree 3 poles (-2.6137, -50.7996) (-2.4799, -50.7123) (-2.1998, -50.5293) (-1.8651, -50.51) (-1.6902, -50.4999) knots 0 0 0 0 0.04708 0.09861 0.09861 0.09861 0.09861
  line L4 (1.9656, -55.6873) -> (1.5636, -55.6873)
  line L5 (1.5636, -55.6873) -> (1.5636, -50.5865)
  line L6 (1.5636, -50.5865) -> (2.1874, -50.5865)
  line L7 (2.1874, -50.5865) -> (2.1874, -54.5611)
  spline S65 degree 3 poles (2.1874, -54.5611) (2.2724, -54.4871) (2.4567, -54.3267) (2.6656, -54.1998) (2.7782, -54.1314) knots 0 0 0 0 0.033753 0.073172 0.073172 0.073172 0.073172
  spline S66 degree 3 poles (2.7782, -54.1314) (2.8925, -54.066) (3.1046, -53.9446) (3.3306, -53.8519) (3.4348, -53.8092) knots 0 0 0 0 0.039461 0.073217 0.073217 0.073217 0.073217
  line L8 (3.4348, -53.8092) -> (3.4348, -54.4121)
  spline S67 degree 3 poles (3.4348, -54.4121) (3.2676, -54.497) (2.9411, -54.6626) (2.6581, -54.8949) (2.52, -55.0081) knots 0 0 0 0 0.056073 0.109474 0.109474 0.109474 0.109474
  spline S68 degree 3 poles (2.52, -55.0081) (2.4022, -55.1179) (2.1861, -55.3192) (2.0345, -55.5723) (1.9656, -55.6873) knots 0 0 0 0 0.048031 0.088061 0.088061 0.088061 0.088061
  line L9 (-4.1821, 49.0969) -> (-2.7891, 52.7769)
  line L10 (-2.7891, 52.7769) -> (-2.2069, 52.7769)
  line L11 (-2.2069, 52.7769) -> (-0.807, 49.0969)
  line L12 (-0.807, 49.0969) -> (-1.4654, 49.0969)
  line L13 (-1.4654, 49.0969) -> (-2.2554, 51.3007)
  spline S69 degree 3 poles (-2.2554, 51.3007) (-2.2975, 51.4217) (-2.3828, 51.6667) (-2.4547, 51.916) (-2.4911, 52.0423) knots 0 0 0 0 0.038408 0.077822 0.077822 0.077822 0.077822
  spline S70 degree 3 poles (-2.4911, 52.0423) (-2.5234, 51.9352) (-2.5946, 51.6998) (-2.6779, 51.4684) (-2.7232, 51.3423) knots 0 0 0 0 0.033566 0.073758 0.073758 0.073758 0.073758
  line L14 (-2.7232, 51.3423) -> (-3.541, 49.0969)
  line L15 (-3.541, 49.0969) -> (-4.1821, 49.0969)
  spline S71 degree 3 poles (1.2687, 52.8601) (1.5111, 52.8423) (1.9804, 52.8079) (2.3427, 52.509) (2.5179, 52.3645) knots 0 0 0 0 0.070957 0.137381 0.137381 0.137381 0.137381
  spline S72 degree 3 poles (2.5179, 52.3645) (2.6566, 52.1699) (2.9595, 51.7448) (2.9821, 51.2209) (2.9944, 50.9369) knots 0 0 0 0 0.070238 0.153394 0.153394 0.153394 0.153394
  spline S73 degree 3 poles (2.9944, 50.9369) (2.9801, 50.6271) (2.954, 50.0574) (2.5915, 49.6215) (2.4261, 49.4226) knots 0 0 0 0 0.090097 0.165714 0.165714 0.165714 0.165714
  spline S74 degree 3 poles (2.4261, 49.4226) (2.2566, 49.3033) (1.9095, 49.0591) (1.4856, 49.0291) (1.2687, 49.0137) knots 0 0 0 0 0.060949 0.124838 0.124838 0.124838 0.124838
  spline S75 degree 3 poles (1.2687, 49.0137) (1.0295, 49.0322) (0.5631, 49.0682) (0.2034, 49.3659) (0.0281, 49.5109) knots 0 0 0 0 0.070069 0.136601 0.136601 0.136601 0.136601
  spline S76 degree 3 poles (0.0281, 49.5109) (-0.1122, 49.701) (-0.4125, 50.1079) (-0.4393, 50.6148) (-0.4535, 50.8849) knots 0 0 0 0 0.069362 0.148467 0.148467 0.148467 0.148467
  spline S77 degree 3 poles (-0.4535, 50.8849) (-0.4494, 51.0992) (-0.4419, 51.4847) (-0.3024, 51.8432) (-0.2404, 52.0024) knots 0 0 0 0 0.06368 0.114552 0.114552 0.114552 0.114552
  spline S78 degree 3 poles (-0.2404, 52.0024) (-0.1611, 52.1307) (-0.0019, 52.3881) (0.2523, 52.5524) (0.3799, 52.6348) knots 0 0 0 0 0.044639 0.089574 0.089574 0.089574 0.089574
  spline S79 degree 3 poles (0.3799, 52.6348) (0.5194, 52.7005) (0.801, 52.8331) (1.1119, 52.851) (1.2687, 52.8601) knots 0 0 0 0 0.045808 0.092453 0.092453 0.092453 0.092453
  line L16 (11.0614, 50.3824) -> (11.0614, 52.7769)
  line L17 (11.0614, 52.7769) -> (11.7336, 52.7769)
  line L18 (11.7336, 52.7769) -> (11.7336, 47.6969)
  line L19 (11.7336, 47.6969) -> (11.0614, 47.6969)
  line L20 (11.0614, 47.6969) -> (11.0614, 49.783)
  line L21 (11.0614, 49.783) -> (8.4209, 49.783)
  line L22 (8.4209, 49.783) -> (8.4209, 47.6969)
  line L23 (8.4209, 47.6969) -> (7.7486, 47.6969)
  line L24 (7.7486, 47.6969) -> (7.7486, 52.7769)
  line L25 (7.7486, 52.7769) -> (8.4209, 52.7769)
  line L26 (8.4209, 52.7769) -> (8.4209, 50.3824)
  line L27 (8.4209, 50.3824) -> (11.0614, 50.3824)
  arc A0 (-52.4404, 15.24) -> (-54.5952, -1.27) centre (0, 0) ccw
  line L28 (-52.4404, 15.24) -> (39.4516, 15.24)
  line L29 (39.4516, 15.24) -> (39.4516, -1.5751)
  line L30 (39.4516, -1.5751) -> (-54.5952, -1.27)
  arc A1 (-27.8243, 46.99) -> (-47.0716, 27.686) centre (0, 0) ccw
  line L31 (-27.8243, 46.99) -> (27.8243, 46.99)
  arc A2 (39.4516, 37.7601) -> (27.8243, 46.99) centre (0, 0) ccw
  line L32 (39.4516, 37.7601) -> (39.4516, 27.686)
  line L33 (39.4516, 27.686) -> (-47.0716, 27.686)
  arc A3 (-50.161, 21.59) -> (-52.0545, 16.51) centre (0, 0) ccw
  line L34 (-50.161, 21.59) -> (39.4516, 21.59)
  line L35 (39.4516, 21.59) -> (39.4516, 16.51)
  line L36 (39.4516, 16.51) -> (-52.0545, 16.51)
  line L37 (39.4516, 26.416) -> (39.4516, 22.86)
  line L38 (39.4516, 22.86) -> (-49.5951, 22.86)
  arc A4 (-47.7959, 26.416) -> (-49.5951, 22.86) centre (0, 0) ccw
  line L39 (-47.7959, 26.416) -> (39.4516, 26.416)
  line L40 (39.4516, -2.8451) -> (39.4516, -37.7601)
  arc A5 (23.0007, -49.53) -> (39.4516, -37.7601) centre (0, 0) ccw
  line L41 (23.0007, -49.53) -> (-23.0007, -49.53)
  arc A6 (-54.5509, -2.5402) -> (-23.0007, -49.53) centre (0, 0) ccw
  line L42 (-54.5509, -2.5402) -> (39.4516, -2.8451)
  circle A7 centre (0, 0) radius 57.15
  line L43 (50.8, -2.54) -> (40.64, -2.54) construction
  line L44 (40.64, -2.54) -> (40.64, -15.24) construction
  line L45 (40.64, -15.24) -> (50.8, -15.24) construction
  line L46 (50.8, -15.24) -> (50.8, -2.54) construction
  line L47 (49.3499, 15.24) -> (40.64, 15.24) construction
  line L48 (40.64, 15.24) -> (40.64, 4.2906) construction
  line L49 (40.64, 4.2906) -> (49.3499, 4.2906) construction
  line L50 (49.3499, 4.2906) -> (49.3499, 15.24) construction
  line L51 (49.2641, 22.86) -> (40.64, 22.86) construction
  line L52 (40.64, 22.86) -> (40.64, 17.9364) construction
  line L53 (40.64, 17.9364) -> (49.2641, 17.9364) construction
  line L54 (49.2641, 17.9364) -> (49.2641, 22.86) construction
  line L55 (48.4595, 30.1179) -> (39.8354, 30.1179) construction
  line L56 (39.8354, 30.1179) -> (39.8354, 25.2984) construction
  line L57 (39.8354, 25.2984) -> (48.4595, 25.2984) construction
  line L58 (48.4595, 25.2984) -> (48.4595, 30.1179) construction
  dimension "d31" = 5.08
  dimension "d32" = 0
  dimension "d33" = 5.08
  dimension "d34" = 0
  dimension "d35" = 5.08
  dimension "d36" = 0
  dimension "d37" = 5.08
  dimension "d38" = 0
  text T0 "20" font "Arial" height 5.08 align centre middle in box 10.16 x 12.7 at (50.8, -2.54) x (-1, 0) y (0, -1) spacing 1
  text T1 "30" font "Arial" height 5.08 align centre middle in box 8.7099 x 10.9494 at (49.3499, 15.24) x (-1, 0) y (0, -1) spacing 1
  text T2 "40" font "Arial" height 5.08 align centre middle in box 8.6241 x 4.9236 at (49.2641, 22.86) x (-1, 0) y (0, -1) spacing 1
  text T3 "50" font "Arial" height 5.08 align centre middle in box 8.6241 x 4.8195 at (48.4595, 30.1179) x (-1, 0) y (0, -1) spacing 1
extrude "Extrude6" cut sketch "Sketch6" against normal blind 1.27 text T3 T2 T1 T0
equation "d23 = 'Hooves'"
equation "d25 = '10'"
equation "d32 = '20'"
equation "d34 = '30'"
equation "d36 = '40'"
equation "d38 = '50'"
